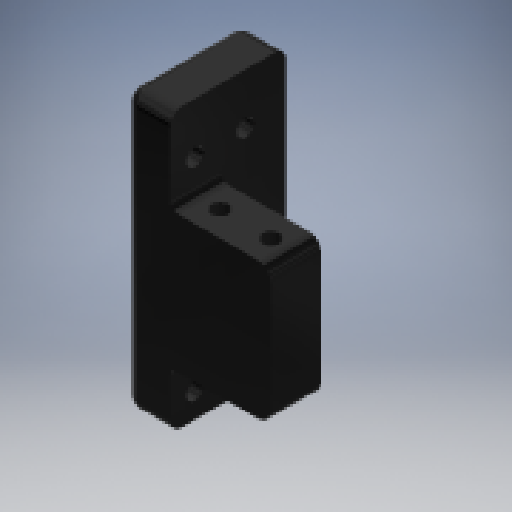
# Autodesk Inventor part: HardStop
Saved by Autodesk Inventor 2026.1 (Build 301233000, 233)
## iProperties
Created: 2025-09-08
Part Number: HardStop
Material: Plastic, Opaque Black
Document SubType Name: Modeling
Designer: Teddy
Density: 0.952 g/cm^3
Appearance: Smooth - Black
Author: Teddy
Autodesk Inventor part; units mm, degrees
ref_plane "YZ Plane" through (0, 0, 0) normal (1, 0, 0) x (0, 1, 0)
ref_plane "XZ Plane" through (0, 0, 0) normal (0, 1, 0) x (-1, 0, 0)
ref_plane "XY Plane" through (0, 0, 0) normal (0, 0, 1) x (1, 0, 0)
ref_plane "Work Plane1" through (22.225, 0, 0) normal (0, 0, 1) x (1, 0, 0)
sketch "Sketch1" plane through (22.225, 0, 0) normal (0, 0, 1) x (1, 0, 0)
  line L0 (-23.8125, 10.8902) -> (-23.8125, 0) projected
  line L1 (-23.8125, -39.6875) -> (-23.8125, -50.5778) projected
  line L2 (-23.8125, 11.9062) -> (-35.2425, 11.9062)
  line L3 (-35.2425, 11.9062) -> (-35.2425, -51.5938)
  line L4 (-35.2425, -51.5938) -> (-23.8125, -51.5938)
  line L5 (-23.8125, -51.5938) -> (-23.8125, 11.9062)
  line L6 (-23.8125, -51.5938) -> (-22.225, -51.5938) projected
  line L7 (-22.225, 11.9062) -> (-23.8125, 11.9062) projected
  point P0 (-22.225, 0)
  point P1 (-23.8125, -50.5778)
  point P2 (-23.8125, 0)
  point P3 (-23.8125, 18.2562)
  dimension "d0" = 11.43
  constraints: 8 end point, 2 coincident, 2 parallel, 1 horizontal, 1 horizontal alignment, 1 perpendicular, 1 point on line
  measures "d0" distance between parallel lines of L5 L3
ref_plane "Work Plane2" through (-1.5875, 3.7528, -29.4386) normal (0, 0, -1) x (0, 1, 0)
extrude "Extrusion1" add sketch "Sketch1" against normal up to surface (29.4386 mm away)
fillet "Fillet1" radius 3.175 2 edges at (-7.3025, -51.5938, -29.4386) (-7.3025, -51.5938, 0)
sketch "Sketch3" plane through (22.225, 0, 0) normal (0, 0, 1) x (1, 0, 0)
  arc A0 (-21.4313, -37.3063) -> (-23.8125, -39.6875) centre (-21.4313, -39.6875) ccw projected
  line L0 (-21.4313, -37.3063) -> (-0.7937, -37.3063) projected
  arc A1 (-23.8125, 0) -> (-21.4313, -2.3813) centre (-21.4313, 0) ccw projected
  line L1 (-13.4239, -2.3813) -> (-21.4313, -2.3813) projected
  line L2 (1.5875, -50.5778) -> (1.5875, -39.6875) projected
  line L3 (1.5875, -39.6875) -> (1.5875, 2.032)
  line L4 (-0.7937, -37.3063) -> (1.5875, -37.3063)
  line L5 (-13.4239, -2.3813) -> (1.5875, -2.3813)
  line L6 (1.5875, -37.0523) -> (-0.7937, -37.0523)
  line L7 (-0.7937, -37.0523) -> (-21.4313, -37.0523)
  arc A2 (-21.4313, -37.0523) -> (-24.0665, -39.6875) centre (-21.4313, -39.6875) ccw
  arc A3 (-24.0665, 0) -> (-21.4313, -2.6353) centre (-21.4313, 0) ccw
  line L8 (-21.4313, -2.6353) -> (-13.4239, -2.6353)
  line L9 (-13.4239, -2.6353) -> (1.5875, -2.6353)
  line L10 (1.5875, -50.5778) -> (7.9375, -50.5778)
  line L11 (7.9375, -50.5778) -> (7.9375, 12.9222)
  line L12 (7.9375, 12.9222) -> (1.5875, 12.9222)
  line L13 (1.5875, 12.9222) -> (1.5875, 2.032)
  arc A4 (-21.4313, -38.8303) -> (-22.2885, -39.6875) centre (-21.4313, -39.6875) ccw
  line L14 (-21.4313, -38.8303) -> (-0.7937, -38.8303)
  line L15 (-0.7937, -38.8303) -> (1.5875, -38.8303)
  line L16 (-22.2885, -39.6875) -> (-22.2885, -48.4188)
  line L17 (-22.2885, -48.4188) -> (-23.8125, -48.4188)
  line L18 (-0.0889, -38.8303) -> (-0.0889, -50.5778)
  line L19 (-0.0889, -50.5778) -> (1.5875, -50.5778)
  line L20 (-23.8125, -51.5938) -> (-22.2885, -51.5938)
  line L21 (-22.2885, -51.5938) -> (-22.2885, -48.4188)
  line L22 (-23.8125, -48.4188) -> (-23.8125, 11.9062) projected
  line L23 (-23.8125, -51.5938) -> (-23.8125, 11.9062)
  point P0 (-22.225, 0)
  point P1 (1.5875, -37.0523)
  point P2 (1.5875, -2.6353)
  point P3 (1.5875, -18.8278)
  point P4 (1.5875, -38.8303)
  point P5 (-23.8125, -1.1288)
  dimension "d6" = 0.254
  dimension "d7" = 0.254
  dimension "d15" = 63.5
  dimension "d16" = 31.75
  dimension "d17" = 6.35
  dimension "d18" = 1.524
  dimension "d19" = 1.6764
  constraints: 40 end point, 8 perpendicular, 6 point on circle, 3 centre point, 3 point on line, 3 vertical, 2 horizontal, 1 collinear, 1 midpoint, 6 other
  measures "d6" distance between parallel lines of L0 L7
  measures "d7" distance between parallel lines of L1 L8
  measures "d15" distance of L10.end L11.end
  measures "d16" distance from line of point (1.588, -18.828) L12
  measures "d17" distance between parallel lines of L3 L11
  measures "d18" radial gap between concentric circles of A0 A4
  measures "d19" distance between parallel lines of L2 L18
extrude "Extrusion3" add sketch "Sketch3" against normal blind 25.4 contours L0 L4 L3 L15 L14 A4 L16 L17 L22 A0 | A0 L22 A2 L7 L6 L3 L4 L0 | L17 L21 L20 L23 | L22 A3 L8 L9 L3 L6 L7 A2 | L3 L13 L12 L11 L10 L2 | L3 L2 L19 L18 L15
fillet "Fillet2" radius 3.175 6 edges at (23.8125, -2.6352, -12.7) (30.1625, 12.9222, -12.7) (30.1625, -50.5778, -12.7) (23.8125, 12.9222, -12.7) (22.1361, -50.5778, -12.7) (22.1361, -38.8303, -12.7)
fillet "Fillet3" radius 3.175 5 edges at (-13.0175, -51.5938, -14.7193) (-0.8255, -51.5938, 0) (-13.0175, 11.9063, -14.7193) (-7.3025, 11.9062, 0) (-7.3025, 11.9063, -29.4386)
sketch "Sketch2" plane through (-13.0175, -51.5938, 0) normal (-1, 0, 0) x (0, 0, 1)
  circle A0 centre (-6.35, 57.15) radius 2.1844 projected
  circle A1 centre (-19.05, 57.15) radius 2.1844 projected
  circle A2 centre (-19.05, 6.35) radius 2.1844 projected
  circle A3 centre (-6.35, 6.35) radius 2.1844 projected
  point P0 (0, 51.5938)
extrude "Extrusion2" cut sketch "Sketch2" against normal blind 43.18 from surface at 0
body "Solid1"
